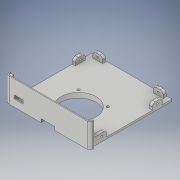
# Autodesk Inventor part: Cover_w_HQcamera
Saved by Autodesk Inventor 2019 (Build 230136000, 136)
## iProperties
Created: 2020-07-04
Part Number: Cover_w_HQcamera
Material: Generic
Document SubType Name: Modeling
Designer: zhang
Density: 1 g/cm^3
Appearance: Default
Author: zhang
Autodesk Inventor part; units mm, degrees
ref_plane "YZ Plane" through (0, 0, 0) normal (1, 0, 0) x (0, 1, 0)
ref_plane "XZ Plane" through (0, 0, 0) normal (0, 1, 0) x (-1, 0, 0)
ref_plane "XY Plane" through (0, 0, 0) normal (0, 0, 1) x (1, 0, 0)
sketch "Sketch1" plane through (0, 0, 0) normal (0, 1, 0) x (-1, 0, 0)
  line L0 (0, 0) -> (-86, 0)
  line L1 (-86, 0) -> (-86, -4)
  line L2 (-86, -4) -> (0, -4)
  line L3 (0, -4) -> (0, 0)
  dimension "d0" = 86
  dimension "d1" = 4
  constraints: 8 end point, 2 parallel, 1 horizontal, 1 perpendicular
  measures "d0" distance of L2.end L1.end
  measures "d1" distance of L1.end L0.end
extrude "Extrusion1" add sketch "Sketch1" along normal blind 25
fillet "Fillet1" radius 3 2 edges at (0, 12.5, 0) (86, 12.5, 0)
sketch "Sketch2" plane through (86, 0, -4) normal (0, 0, -1) x (-1, 0, 0)
  line L0 (0, 25) -> (80, 25)
  line L1 (0.95, 25) -> (85.05, 25)
  line L2 (85.05, 25) -> (85.05, 24.25)
  line L3 (85.05, 24.25) -> (0.95, 24.25)
  line L4 (0.95, 24.25) -> (0.95, 25)
  line L5 (86, 0) -> (86, 25)
  line L6 (3.95, 24.25) -> (82.05, 24.25)
  line L7 (82.05, 24.25) -> (82.05, 22.5)
  line L8 (82.05, 22.5) -> (3.95, 22.5)
  line L9 (3.95, 22.5) -> (3.95, 24.25)
  line L10 (0.95, 22.5) -> (85.05, 22.5)
  line L11 (85.05, 22.5) -> (85.05, 20.7)
  line L12 (85.05, 20.7) -> (0.95, 20.7)
  line L13 (0.95, 20.7) -> (0.95, 22.5)
  line L14 (2, 20.7) -> (84, 20.7)
  line L15 (84, 20.7) -> (84, 2)
  line L16 (84, 2) -> (2, 2)
  line L17 (2, 2) -> (2, 20.7)
  line L18 (0, 0) -> (80, 0)
  line L19 (0, 0) -> (0, 25)
  line L20 (86, 0) -> (86, 25) projected
  line L21 (0, 0) -> (86, 0) projected
  line L22 (0, 25) -> (86, 25) projected
  line L23 (0, 0) -> (0, 25) projected
  dimension "d5" = 0.75
  dimension "d6" = 84.1
  dimension "d7" = 0.95
  dimension "d8" = 1.75
  dimension "d9" = 3
  dimension "d10" = 3
  dimension "d11" = 1.8
  dimension "d12" = 2
  dimension "d13" = 2
  dimension "d14" = 2
  dimension "d15" = 25
  constraints: 40 end point, 8 parallel, 6 collinear, 4 horizontal, 4 perpendicular, 4 point on line
  measures "d5" distance of L1.end L2.end
  measures "d6" distance of L2.end L3.end
  measures "d7" distance between parallel lines of L5 L2
  measures "d8" distance of L6.end L7.end
  measures "d9" distance between parallel lines of L9 L4
  measures "d10" distance between parallel lines of L2 L7
  measures "d11" distance of L12.end L10.start
  measures "d12" distance between parallel lines of L18 L16
  measures "d13" distance between parallel lines of L19 L17
  measures "d14" distance between parallel lines of L5 L15
  measures "d15" distance of L19.start L19.end
extrude "Extrusion2" cut sketch "Sketch2" against normal blind 3 contours L0 L1 L2 L3 L4 | L3 L7 L8 L9 | L8 L10 L11 L12 L13 | L12 L15 L16 L17
fillet "Fillet2" radius 2 2 edges at (0.95, 24.625, -1) (85.05, 24.625, -1)
sketch "Sketch3" plane through (86, 0, -4) normal (0, 0, -1) x (-1, 0, 0)
  line L0 (84, 2) -> (2, 2) projected
  line L1 (0, 0) -> (86, 0) projected
  line L2 (2, 2) -> (84, 2)
  line L3 (84, 2) -> (84, 0)
  line L4 (84, 0) -> (2, 0)
  line L5 (2, 0) -> (2, 2)
  line L6 (84, 20.7) -> (84, 2) projected
  constraints: 8 end point, 2 parallel, 1 collinear, 1 horizontal, 1 perpendicular, 1 point on line
extrude "Extrusion3" add sketch "Sketch3" along normal blind 82
sketch "Sketch4" plane through (2, 2, -1) normal (0, 1, 0) x (1, 0, 0)
  line L0 (1, -1) -> (81, -1) projected
  line L1 (-2, 3) -> (-2, 2) projected
  line L2 (22, 49.25) -> (60, 49.25)
  line L3 (60, 49.25) -> (60, 11.25)
  line L4 (60, 11.25) -> (22, 11.25)
  line L5 (22, 11.25) -> (22, 49.25)
  point P0 (-2, -1)
  dimension "d25" = 38
  dimension "d26" = 38
  dimension "d27" = 12.25
  dimension "d28" = 24
  constraints: 8 end point, 2 parallel, 1 horizontal, 1 perpendicular
  measures "d25" distance of L3.end L4.end
  measures "d26" distance of L2.end L3.end
  measures "d27" distance between parallel lines of L0 L4
  measures "d28" distance between parallel lines of L1 L5
extrude "Extrusion4" add sketch "Sketch4" against normal blind 5
sketch "Sketch5" plane through (2, -3, -1) normal (0, -1, 0) x (1, 0, 0)
  circle A0 centre (41, -30.25) radius 18
  line L0 (22, -11.25) -> (22, -49.25) projected
  line L1 (60, -11.25) -> (22, -11.25) projected
  line L2 (48.05, -20) -> (33.95, -20)
  line L3 (33.95, -20) -> (33.95, 1)
  line L4 (33.95, 1) -> (48.05, 1)
  line L5 (48.05, 1) -> (48.05, -20)
  line L6 (1, 1) -> (81, 1) projected
  line L7 (0, 0) -> (82, 0) projected
  line L8 (53.5, -17.5) -> (28.5, -17.5)
  line L9 (28.5, -17.5) -> (28.5, -5.5)
  line L10 (28.5, -5.5) -> (53.5, -5.5)
  line L11 (53.5, -5.5) -> (53.5, -17.5)
  line L12 (60, -49.25) -> (60, -11.25) projected
  point P0 (-2, 1)
  dimension "d31" = 36
  dimension "d32" = 19
  dimension "d33" = 19
  dimension "d34" = 14.1
  dimension "d35" = 11.95
  dimension "d36" = 20
  dimension "d37" = 25
  dimension "d38" = 12
  dimension "d39" = 6.5
  dimension "d40" = 6.5
  constraints: 16 end point, 4 parallel, 2 horizontal, 2 perpendicular, 1 centre point, 1 collinear
  measures "d31" diameter of A0
  measures "d32" distance from line of L0 A0.centre
  measures "d33" distance from line of L1 A0.centre
  measures "d34" distance of L2.start L2.end
  measures "d35" distance between parallel lines of L0 L3
  measures "d36" distance between parallel lines of L7 L2
  measures "d37" distance of L9.end L10.end
  measures "d38" distance of L8.end L9.end
  measures "d39" distance between parallel lines of L12 L11
  measures "d40" distance between parallel lines of L4 L10
extrude "Extrusion5" cut sketch "Sketch5" against normal blind 6.5
sketch "Sketch6" plane through (2, -3, -1) normal (0, -1, 0) x (1, 0, 0)
  circle A0 centre (56, -45.25) radius 1.3
  circle A1 centre (26, -45.25) radius 1.3
  circle A2 centre (56, -15.25) radius 1.3
  circle A3 centre (26, -15.25) radius 1.3
  line L0 (22, -49.25) -> (60, -49.25) projected
  line L1 (60, -49.25) -> (60, -11.25) projected
  line L2 (22, -11.25) -> (22, -49.25) projected
  line L3 (60, -11.25) -> (53.5, -11.25) projected
  line L4 (28.5, -11.25) -> (22, -11.25) projected
  point P0 (-2, 1)
  dimension "d43" = 2.6
  dimension "d44" = 2.6
  dimension "d45" = 2.6
  dimension "d46" = 2.6
  dimension "d47" = 4
  dimension "d48" = 4
  dimension "d49" = 4
  dimension "d50" = 4
  dimension "d51" = 4
  dimension "d52" = 4
  dimension "d53" = 4
  dimension "d54" = 4
  constraints: 4 centre point
  measures "d43" diameter of A0
  measures "d44" diameter of A1
  measures "d45" diameter of A2
  measures "d46" diameter of A3
  measures "d47" distance from line of A0.centre L0
  measures "d48" distance from line of L1 A0.centre
  measures "d49" distance from line of L2 A1.centre
  measures "d50" distance from line of L0 A1.centre
  measures "d51" distance from line of L3 A2.centre
  measures "d52" distance from line of L1 A2.centre
  measures "d53" distance from line of L2 A3.centre
  measures "d54" distance from line of L4 A3.centre
extrude "Extrusion6" cut sketch "Sketch6" against normal blind 12.5
sketch "Sketch7" plane through (2, -3, -1) normal (0, -1, 0) x (1, 0, 0)
  circle A0 centre (56, -45.25) radius 1.3 projected
  line L0 (53.5, -43.8066) -> (56, -42.3632)
  line L1 (56, -42.3632) -> (58.5, -43.8066)
  line L2 (58.5, -43.8066) -> (58.5, -46.6934)
  line L3 (58.5, -46.6934) -> (56, -48.1368)
  line L4 (56, -48.1368) -> (53.5, -46.6934)
  line L5 (53.5, -46.6934) -> (53.5, -43.8066)
  circle A1 centre (26, -45.25) radius 1.3 projected
  line L6 (23.5, -43.8066) -> (26, -42.3632)
  line L7 (26, -42.3632) -> (28.5, -43.8066)
  line L8 (28.5, -43.8066) -> (28.5, -46.6934)
  line L9 (28.5, -46.6934) -> (26, -48.1368)
  line L10 (26, -48.1368) -> (23.5, -46.6934)
  line L11 (23.5, -46.6934) -> (23.5, -43.8066)
  circle A2 centre (26, -15.25) radius 1.3 projected
  line L12 (23.5, -13.8066) -> (26, -12.3632)
  line L13 (26, -12.3632) -> (28.5, -13.8066)
  line L14 (28.5, -13.8066) -> (28.5, -16.6934)
  line L15 (28.5, -16.6934) -> (26, -18.1368)
  line L16 (26, -18.1368) -> (23.5, -16.6934)
  line L17 (23.5, -16.6934) -> (23.5, -13.8066)
  circle A3 centre (56, -15.25) radius 1.3 projected
  line L18 (53.5, -16.6934) -> (53.5, -13.8066)
  line L19 (53.5, -13.8066) -> (56, -12.3632)
  line L20 (56, -12.3632) -> (58.5, -13.8066)
  line L21 (58.5, -13.8066) -> (58.5, -16.6934)
  line L22 (58.5, -16.6934) -> (56, -18.1368)
  line L23 (56, -18.1368) -> (53.5, -16.6934)
  line L24 (22, -11.25) -> (22, -49.25) projected
  line L25 (60, -49.25) -> (60, -11.25) projected
  point P0 (-2, 1)
  dimension "d57" = 5
  dimension "d58" = 5
  dimension "d59" = 5
  dimension "d60" = 5
  constraints: 48 end point, 4 coincident, 4 parallel, 52 other
  measures "d57" distance between parallel lines of L17 L14
  measures "d58" distance between parallel lines of L22 L19
  measures "d59" distance between parallel lines of L5 L2
  measures "d60" distance between parallel lines of L11 L8
extrude "Extrusion7" cut sketch "Sketch7" against normal blind 2
sketch "Sketch8" plane through (0, 0, 0) normal (0, -1, 0) x (1, 0, 0)
  line L0 (79, -85) -> (69, -85)
  line L1 (69, -85) -> (69, -82)
  line L2 (69, -82) -> (79, -82)
  line L3 (79, -82) -> (79, -85)
  line L4 (17, -85) -> (7, -85)
  line L5 (7, -85) -> (7, -82)
  line L6 (7, -82) -> (17, -82)
  line L7 (17, -82) -> (17, -85)
  line L8 (84, -4) -> (84, -86) projected
  line L9 (2, -4) -> (2, -86) projected
  line L10 (84, -86) -> (2, -86) projected
  point P0 (0, 0)
  dimension "d63" = 10
  dimension "d64" = 10
  dimension "d65" = 3
  dimension "d66" = 3
  dimension "d67" = 5
  dimension "d68" = 5
  dimension "d69" = 1
  constraints: 16 end point, 4 parallel, 2 horizontal, 2 perpendicular, 1 point on line
  measures "d63" distance of L1.end L2.end
  measures "d64" distance of L5.end L6.end
  measures "d65" distance of L4.end L5.end
  measures "d66" distance of L0.end L1.end
  measures "d67" distance between parallel lines of L8 L3
  measures "d68" distance between parallel lines of L9 L5
  measures "d69" distance between parallel lines of L10 L0
extrude "Extrusion8" add sketch "Sketch8" against normal blind 8
fillet "Fillet3" radius 3 4 edges at (79, 8, -83.5) (69, 8, -83.5) (17, 8, -83.5) (7, 8, -83.5)
sketch "Sketch9" plane through (79, 2, -85) normal (0, 0, -1) x (-1, 0, 0)
  circle A0 centre (5, 3) radius 1
  circle A1 centre (67, 3) radius 1
  line L0 (-5, -2) -> (77, -2) projected
  line L1 (-5, 0) -> (-5, -2) projected
  point P0 (79, -2)
  point P1 (77, 0)
  dimension "d72" = 2
  dimension "d73" = 2
  dimension "d74" = 5
  dimension "d75" = 5
  dimension "d76" = 10
  dimension "d77" = 10
  constraints: 2 centre point
  measures "d72" diameter of A0
  measures "d73" diameter of A1
  measures "d74" distance from line of L0 A0.centre
  measures "d75" distance from line of L0 A1.centre
  measures "d76" horizontal distance of point (77, 0) A1.centre
  measures "d77" distance from line of L1 A0.centre
extrude "Extrusion9" cut sketch "Sketch9" against normal blind 8
sketch "Sketch10" plane through (86, 0, -1) normal (0, 0, -1) x (-1, 0, 0)
  line L0 (2, 2) -> (2, 20.7) projected
  line L1 (2, 8) -> (5, 8)
  line L2 (5, 8) -> (5, 2)
  line L3 (5, 2) -> (2, 2)
  line L4 (2, 2) -> (2, 8)
  line L5 (84, 20.7) -> (84, 2) projected
  line L6 (84, 8) -> (81, 8)
  line L7 (81, 8) -> (81, 2)
  line L8 (81, 2) -> (84, 2)
  line L9 (84, 2) -> (84, 8)
  line L10 (2, 0) -> (84, 0) projected
  line L11 (84, 2) -> (2, 2) projected
  point P0 (86, 0)
  dimension "d81" = 3
  dimension "d82" = 6
  dimension "d83" = 3
  dimension "d84" = 6
  constraints: 16 end point, 4 parallel, 2 collinear, 2 horizontal, 2 perpendicular, 2 point on line
  measures "d81" distance of L2.end L3.end
  measures "d82" distance of L1.end L2.end
  measures "d83" distance of L8.end L7.end
  measures "d84" distance of L7.end L6.end
extrude "Extrusion10" add sketch "Sketch10" along normal blind 18
fillet "Fillet4" radius 3 2 edges at (82.5, 8, -19) (3.5, 8, -19)
sketch "Sketch12" plane through (84, 0, -86) normal (1, 0, 0) x (0, 0, -1)
  circle A0 centre (-72, 5) radius 1
  line L0 (-82, 0) -> (0, 0) projected
  line L1 (-82, 0) -> (-82, 25) projected
  point P0 (-86, 0)
  dimension "d98" = 2
  dimension "d99" = 5
  dimension "d100" = 10
  constraints: 1 centre point
  measures "d98" diameter of A0
  measures "d99" distance from line of L0 A0.centre
  measures "d100" distance from line of L1 A0.centre
fillet "Fillet5" radius 2 2 edges at (0.95, 21.6, -1) (85.05, 21.6, -1)
extrude "Extrusion12" cut sketch "Sketch12" against normal through all
sketch "Sketch13" plane through (2, 2, -86) normal (0, 1, 0) x (1, 0, 0)
  line L0 (0, -67) -> (0, 0) projected
  line L1 (0, -20) -> (3, -20)
  line L2 (3, -20) -> (3, -10)
  line L3 (3, -10) -> (0, -10)
  line L4 (0, -10) -> (0, -20)
  line L5 (82, -67) -> (82, 0) projected
  line L6 (82, -20) -> (79, -20)
  line L7 (79, -20) -> (79, -10)
  line L8 (79, -10) -> (82, -10)
  line L9 (82, -10) -> (82, -20)
  line L10 (0, 0) -> (82, 0) projected
  point P0 (-2, -86)
  dimension "d103" = 3
  dimension "d104" = 10
  dimension "d105" = 3
  dimension "d106" = 10
  dimension "d107" = 10
  dimension "d108" = 10
  constraints: 16 end point, 4 parallel, 2 horizontal, 2 perpendicular, 2 point on line
  measures "d103" distance of L3.end L2.end
  measures "d104" distance of L2.end L1.end
  measures "d105" distance of L7.end L8.end
  measures "d106" distance of L6.end L7.end
  measures "d107" distance between parallel lines of L10 L3
  measures "d108" distance between parallel lines of L8 L10
extrude "Extrusion13" add sketch "Sketch13" along normal blind 6
fillet "Fillet6" radius 3 4 edges at (82.5, 8, -66) (82.5, 8, -76) (3.5, 8, -66) (3.5, 8, -76)
sketch "Sketch14" plane through (84, 0, -86) normal (1, 0, 0) x (0, 0, -1)
  circle A0 centre (-15, 5) radius 1
  line L0 (-82, 0) -> (0, 0) projected
  line L1 (0, 2) -> (0, 0) projected
  point P0 (-86, 0)
  dimension "d112" = 2
  dimension "d113" = 5
  dimension "d114" = 15
  constraints: 1 centre point
  measures "d112" diameter of A0
  measures "d113" distance from line of L0 A0.centre
  measures "d114" distance from line of L1 A0.centre
extrude "Extrusion14" cut sketch "Sketch14" against normal through all
sketch "Sketch16" plane through (86, 0, -1) normal (0, 0, -1) x (-1, 0, 0)
  line L0 (77.5, 7.5) -> (68.5, 7.5)
  line L1 (68.5, 7.5) -> (68.5, 11)
  line L2 (68.5, 11) -> (77.5, 11)
  line L3 (77.5, 11) -> (77.5, 7.5)
  line L4 (85.05, 25) -> (86, 25) projected
  line L5 (86, 0) -> (86, 25) projected
  line L6 (83, 0) -> (50.05, 0) projected
  line L7 (71.7526, 7.5) -> (80.9554, 7.5)
  line L8 (80.9554, 7.5) -> (80.9554, 0)
  line L9 (80.9554, 0) -> (71.7526, 0)
  line L10 (71.7526, 0) -> (71.7526, 7.5)
  dimension "d120" = 9
  dimension "d121" = 3.5
  dimension "d123" = 17.5
  dimension "d126" = 7.5
  constraints: 16 end point, 4 parallel, 2 horizontal, 2 perpendicular, 2 point on line
  measures "d120" distance of L1.end L2.end
  measures "d121" distance of L0.end L1.end
  measures "d123" distance between parallel lines of L1 L5
  measures "d126" distance between parallel lines of L6 L0
extrude "Extrusion15" cut sketch "Sketch16" against normal blind 5 contours L0 L1 L2 L3
body "Solid1"
